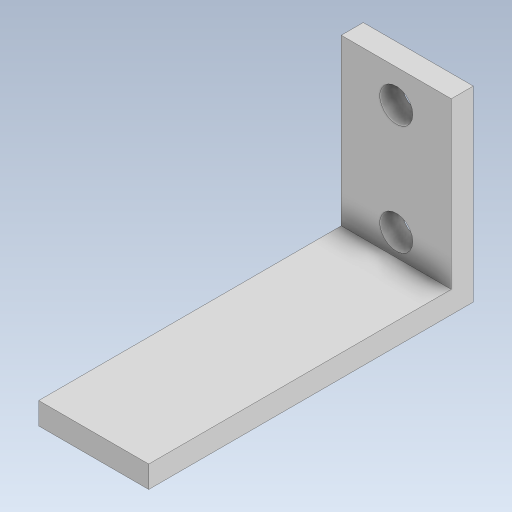
# Autodesk Inventor part: Bracket Lifter Motor 2
Saved by Autodesk Inventor 2023.5 (Build 275446000, 446)
## iProperties
Created: 2025-09-27
Part Number: Bracket Lifter Motor 2
Material: Generic
Document SubType Name: Modeling
Designer: Guntur
Density: 1 g/cm^3
Appearance: Default
Author: Guntur
Autodesk Inventor part; units mm, degrees
ref_plane "YZ Plane" through (0, 0, 0) normal (1, 0, 0) x (0, 1, 0)
ref_plane "XZ Plane" through (0, 0, 0) normal (0, 1, 0) x (-1, 0, 0)
ref_plane "XY Plane" through (0, 0, 0) normal (0, 0, 1) x (1, 0, 0)
sketch "Sketch1" plane through (0, 0, 0) normal (0, 1, 0) x (-1, 0, 0)
  line L0 (5, 14.75) -> (-5, 14.75)
  line L1 (-5, 14.75) -> (-5, -14.75)
  line L2 (-5, -14.75) -> (5, -14.75)
  line L3 (5, -14.75) -> (5, 14.75)
  line L4 (5, 14.75) -> (-5, -14.75) construction
  line L5 (-5, 14.75) -> (5, -14.75) construction
  point P0 (0, 0)
  dimension "d0" = 10
  dimension "d1" = 29.5
  constraints: 12 end point, 2 midpoint, 2 parallel, 1 horizontal, 1 perpendicular
  measures "d0" distance of L2.end L1.end
  measures "d1" distance of L1.end L0.end
extrude "Extrusion1" add sketch "Sketch1" along normal blind 2
sketch "Sketch2" plane through (0, 2, 0) normal (0, 1, 0) x (1, 0, 0)
  line L0 (5, 14.75) -> (-5, 14.75) projected
  line L1 (5, -14.75) -> (5, 14.75) projected
  line L2 (-5, 14.75) -> (5, 14.75)
  line L3 (5, 14.75) -> (5, 12.75)
  line L4 (5, 12.75) -> (-5, 12.75)
  line L5 (-5, 12.75) -> (-5, 14.75)
  point P0 (0, 0)
  dimension "d4" = 2
  constraints: 8 end point, 2 parallel, 1 horizontal, 1 perpendicular, 1 point on line
  measures "d4" distance of L2.end L3.end
extrude "Extrusion2" add sketch "Sketch2" along normal blind 15
sketch "Sketch3" plane through (-5, 2, -12.75) normal (0, 0, 1) x (1, 0, 0)
  circle A0 centre (5, 12) radius 1.5
  circle A1 centre (5, 2) radius 1.5
  line L0 (0, 0) -> (10, 0) projected
  point P0 (5, -2)
  dimension "d7" = 3
  dimension "d8" = 3
  dimension "d9" = 2
  dimension "d10" = 10
  constraints: 2 centre point
  measures "d7" diameter of A0
  measures "d8" diameter of A1
  measures "d9" distance from line of L0 A1.centre
  measures "d10" distance of A1.centre A0.centre
extrude "Extrusion3" cut sketch "Sketch3" against normal blind 15
body "Solid1"
